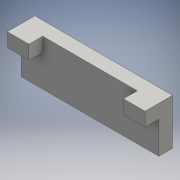
# Autodesk Inventor part: Tirador
Saved by Autodesk Inventor 2016 (Build 200138000, 138)
## iProperties
Created: 2015-08-31
Part Number: Tirador
Material: Generic
Document SubType Name: Modeling
Designer: amatiasq
Density: 1 g/cm^3
Appearance: Default
Author: amatiasq
Autodesk Inventor part; units mm, degrees
ref_plane "YZ Plane" through (0, 0, 0) normal (1, 0, 0) x (0, 1, 0)
ref_plane "XZ Plane" through (0, 0, 0) normal (0, 1, 0) x (-1, 0, 0)
ref_plane "XY Plane" through (0, 0, 0) normal (0, 0, 1) x (1, 0, 0)
sketch "Sketch1" plane through (0, 0, 0) normal (0, 1, 0) x (-1, 0, 0)
  line L0 (0, 0) -> (-30, 0)
  line L1 (-30, 0) -> (-30, -10)
  line L2 (-30, -10) -> (0, -10)
  line L3 (0, -10) -> (0, 0)
  dimension "d0" = 30
  dimension "d1" = 10
  constraints: 8 end point, 2 parallel, 1 horizontal, 1 perpendicular
  measures "d0" distance of L2.end L1.end
  measures "d1" distance between parallel lines of L2 L0
extrude "Cuerpo" add sketch "Sketch1" against normal blind 3
sketch "Sketch2" plane through (0, -3, 0) normal (0, -1, 0) x (1, 0, 0)
  line L0 (30, 0) -> (25.3, 0)
  line L1 (25.3, 0) -> (25.3, -3)
  line L2 (25.3, -3) -> (30, -3)
  line L3 (30, -3) -> (30, 0)
  line L4 (0, 0) -> (4.7, 0)
  line L5 (4.7, 0) -> (4.7, -3)
  line L6 (4.7, -3) -> (0, -3)
  line L7 (0, -3) -> (0, 0)
  dimension "d4" = 4.7
  dimension "d5" = 3
  dimension "d6" = 3
  dimension "d7" = 4.7
  constraints: 16 end point, 4 parallel, 2 coincident, 2 horizontal, 2 perpendicular
  measures "d4" distance between parallel lines of L1 L3
  measures "d5" distance between parallel lines of L2 L0
  measures "d6" distance between parallel lines of L6 L4
  measures "d7" distance between parallel lines of L5 L7
extrude "Agarres" add sketch "Sketch2" along normal blind 3
equation "\"d0\" = hoja_ancho_total"
equation "\"d1\" = tirador_largo"
equation "\"d2\" = deslizador_alto"
equation "\"d4\" = hoja_stop_saliente - margen"
equation "\"d5\" = tirador_agarre_largo"
equation "\"d6\" = d5"
equation "\"d7\" = d4"
equation "\"d8\" = hoja_alto"
equation "\"base_alto\" = 3"
equation "\"hoja_alto\" = 3"
equation "\"hoja_cola_biselado\" = 1"
equation "\"hoja_filo_biselado\" = 0.5"
equation "\"hoja_stop_biselado\" = 2"
equation "\"hoja_stop_largo\" = 5"
equation "\"hoja_stop_posicion\" = 5"
equation "\"hoja_stop_saliente\" = 5"
equation "\"margen\" = 0.3"
equation "\"muros_grosor\" = 3"
equation "\"rail_alto\" = 1.5"
equation "\"rail_grosor\" = 5"
equation "\"hoja_ancho_total\" = 30"
equation "\"deslizador_soporte_ancho\" = 5"
equation "\"deslizador_soporte_alto\" = 5"
equation "\"deslizador_tope_alto\" = 5"
equation "\"deslizador_alto\" = 3"
equation "\"tirador_agarre_largo\" = 3"
equation "\"tirador_largo\" = 10"
body "Solid1"
